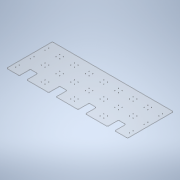
# Autodesk Inventor part: CC-bottomPlate
Saved by Autodesk Inventor 2020 (Build 240168000, 168)
## iProperties
Created: 2019-05-04
Part Number: CC-bottomPlate
Material: Polycarbonate, Clear
Document SubType Name: Modeling
Designer: andwh
Density: 1.2 g/cm^3
Appearance: Polycarbonate - Clear
Author: andwh
Autodesk Inventor part; units mm, degrees
ref_plane "YZ Plane" through (0, 0, 0) normal (1, 0, 0) x (0, 1, 0)
ref_plane "XZ Plane" through (0, 0, 0) normal (0, 1, 0) x (-1, 0, 0)
ref_plane "XY Plane" through (0, 0, 0) normal (0, 0, 1) x (1, 0, 0)
sketch "Sketch1" plane through (0, 0, 0) normal (0, 1, 0) x (-1, 0, 0)
  line L0 (0, 0) -> (-838.2, 0)
  line L1 (-838.2, 0) -> (-838.2, -317.5)
  line L2 (-838.2, -317.5) -> (0, -317.5)
  line L3 (0, -317.5) -> (0, 0)
  circle A0 centre (-63.5, -50.8) radius 44.45 construction
  circle A1 centre (-25.4, -63.5) radius 2.0193
  circle A2 centre (-101.6, -63.5) radius 2.0193
  circle A3 centre (-25.4, -38.1) radius 2.0193
  circle A4 centre (-101.6, -38.1) radius 2.0193
  circle A5 centre (-63.5, -50.8) radius 1.27 construction
  circle A6 centre (-127, -38.1) radius 2.0193
  circle A7 centre (-127, -63.5) radius 2.0193
  circle A8 centre (-165.1, -50.8) radius 1.27 construction
  circle A9 centre (-203.2, -63.5) radius 2.0193
  circle A10 centre (-203.2, -38.1) radius 2.0193
  circle A11 centre (-228.6, -38.1) radius 2.0193
  circle A12 centre (-228.6, -63.5) radius 2.0193
  circle A13 centre (-266.7, -50.8) radius 1.27 construction
  circle A14 centre (-304.8, -63.5) radius 2.0193
  circle A15 centre (-304.8, -38.1) radius 2.0193
  circle A16 centre (-330.2, -38.1) radius 2.0193
  circle A17 centre (-330.2, -63.5) radius 2.0193
  circle A18 centre (-368.3, -50.8) radius 1.27 construction
  circle A19 centre (-406.4, -63.5) radius 2.0193
  circle A20 centre (-406.4, -38.1) radius 2.0193
  circle A21 centre (-431.8, -38.1) radius 2.0193
  circle A22 centre (-431.8, -63.5) radius 2.0193
  circle A23 centre (-469.9, -50.8) radius 1.27 construction
  circle A24 centre (-508, -63.5) radius 2.0193
  circle A25 centre (-508, -38.1) radius 2.0193
  circle A26 centre (-533.4, -38.1) radius 2.0193
  circle A27 centre (-533.4, -63.5) radius 2.0193
  circle A28 centre (-571.5, -50.8) radius 1.27 construction
  circle A29 centre (-609.6, -63.5) radius 2.0193
  circle A30 centre (-609.6, -38.1) radius 2.0193
  circle A31 centre (-635, -38.1) radius 2.0193
  circle A32 centre (-635, -63.5) radius 2.0193
  circle A33 centre (-673.1, -50.8) radius 1.27 construction
  circle A34 centre (-711.2, -63.5) radius 2.0193
  circle A35 centre (-711.2, -38.1) radius 2.0193
  circle A36 centre (-736.6, -38.1) radius 2.0193
  circle A37 centre (-736.6, -63.5) radius 2.0193
  circle A38 centre (-774.7, -50.8) radius 1.27 construction
  circle A39 centre (-812.8, -63.5) radius 2.0193
  circle A40 centre (-812.8, -38.1) radius 2.0193
  circle A41 centre (-25.4, -139.7) radius 2.0193
  circle A42 centre (-25.4, -165.1) radius 2.0193
  circle A43 centre (-63.5, -152.4) radius 1.27 construction
  circle A44 centre (-101.6, -165.1) radius 2.0193
  circle A45 centre (-101.6, -139.7) radius 2.0193
  circle A46 centre (-127, -139.7) radius 2.0193
  circle A47 centre (-127, -165.1) radius 2.0193
  circle A48 centre (-165.1, -152.4) radius 1.27 construction
  circle A49 centre (-203.2, -165.1) radius 2.0193
  circle A50 centre (-203.2, -139.7) radius 2.0193
  circle A51 centre (-228.6, -139.7) radius 2.0193
  circle A52 centre (-228.6, -165.1) radius 2.0193
  circle A53 centre (-266.7, -152.4) radius 1.27 construction
  circle A54 centre (-304.8, -165.1) radius 2.0193
  circle A55 centre (-304.8, -139.7) radius 2.0193
  circle A56 centre (-330.2, -139.7) radius 2.0193
  circle A57 centre (-330.2, -165.1) radius 2.0193
  circle A58 centre (-368.3, -152.4) radius 1.27 construction
  circle A59 centre (-406.4, -165.1) radius 2.0193
  circle A60 centre (-406.4, -139.7) radius 2.0193
  circle A61 centre (-431.8, -139.7) radius 2.0193
  circle A62 centre (-431.8, -165.1) radius 2.0193
  circle A63 centre (-469.9, -152.4) radius 1.27 construction
  circle A64 centre (-508, -165.1) radius 2.0193
  circle A65 centre (-508, -139.7) radius 2.0193
  circle A66 centre (-533.4, -139.7) radius 2.0193
  circle A67 centre (-533.4, -165.1) radius 2.0193
  circle A68 centre (-571.5, -152.4) radius 1.27 construction
  circle A69 centre (-609.6, -165.1) radius 2.0193
  circle A70 centre (-609.6, -139.7) radius 2.0193
  circle A71 centre (-635, -139.7) radius 2.0193
  circle A72 centre (-635, -165.1) radius 2.0193
  circle A73 centre (-673.1, -152.4) radius 1.27 construction
  circle A74 centre (-711.2, -165.1) radius 2.0193
  circle A75 centre (-711.2, -139.7) radius 2.0193
  circle A76 centre (-736.6, -139.7) radius 2.0193
  circle A77 centre (-736.6, -165.1) radius 2.0193
  circle A78 centre (-774.7, -152.4) radius 1.27 construction
  circle A79 centre (-812.8, -165.1) radius 2.0193
  circle A80 centre (-812.8, -139.7) radius 2.0193
  circle A81 centre (-25.4, -241.3) radius 2.0193
  circle A82 centre (-25.4, -266.7) radius 2.0193
  circle A83 centre (-63.5, -254) radius 1.27 construction
  circle A84 centre (-101.6, -266.7) radius 2.0193
  circle A85 centre (-101.6, -241.3) radius 2.0193
  circle A86 centre (-127, -241.3) radius 2.0193
  circle A87 centre (-127, -266.7) radius 2.0193
  circle A88 centre (-165.1, -254) radius 1.27 construction
  circle A89 centre (-203.2, -266.7) radius 2.0193
  circle A90 centre (-203.2, -241.3) radius 2.0193
  circle A91 centre (-228.6, -241.3) radius 2.0193
  circle A92 centre (-228.6, -266.7) radius 2.0193
  circle A93 centre (-266.7, -254) radius 1.27 construction
  circle A94 centre (-304.8, -266.7) radius 2.0193
  circle A95 centre (-304.8, -241.3) radius 2.0193
  circle A96 centre (-330.2, -241.3) radius 2.0193
  circle A97 centre (-330.2, -266.7) radius 2.0193
  circle A98 centre (-368.3, -254) radius 1.27 construction
  circle A99 centre (-406.4, -266.7) radius 2.0193
  circle A100 centre (-406.4, -241.3) radius 2.0193
  circle A101 centre (-431.8, -241.3) radius 2.0193
  circle A102 centre (-431.8, -266.7) radius 2.0193
  circle A103 centre (-469.9, -254) radius 1.27 construction
  circle A104 centre (-508, -266.7) radius 2.0193
  circle A105 centre (-508, -241.3) radius 2.0193
  circle A106 centre (-533.4, -241.3) radius 2.0193
  circle A107 centre (-533.4, -266.7) radius 2.0193
  circle A108 centre (-571.5, -254) radius 1.27 construction
  circle A109 centre (-609.6, -266.7) radius 2.0193
  circle A110 centre (-609.6, -241.3) radius 2.0193
  circle A111 centre (-635, -241.3) radius 2.0193
  circle A112 centre (-635, -266.7) radius 2.0193
  circle A113 centre (-673.1, -254) radius 1.27 construction
  circle A114 centre (-711.2, -266.7) radius 2.0193
  circle A115 centre (-711.2, -241.3) radius 2.0193
  circle A116 centre (-736.6, -241.3) radius 2.0193
  circle A117 centre (-736.6, -266.7) radius 2.0193
  circle A118 centre (-774.7, -254) radius 1.27 construction
  circle A119 centre (-812.8, -266.7) radius 2.0193
  circle A120 centre (-812.8, -241.3) radius 2.0193
  dimension "d2" = 88.9
  dimension "d3" = 63.5
  dimension "d4" = 50.8
  dimension "d15" = 838.2
  dimension "d16" = 317.5
  dimension "d44" = 4.0386
  dimension "d49" = 76.2
  dimension "d52" = 25.4
  dimension "d126" = 12.7
  dimension "d127" = 38.1
  dimension "d130" = 101.6
  dimension "d133" = 101.6
  dimension "d153" = 63.5
  dimension "d154" = 2.54
  constraints: 121 centre point, 8 end point, 3 horizontal, 2 parallel, 2 vertical, 1 coincident, 1 perpendicular, 236 other
  measures "d2" diameter of A0
  measures "d3" distance from line of L3 A0.centre
  measures "d4" distance from line of L0 A0.centre
  measures "d15" distance of L1.end L2.end
  measures "d16" distance of L0.end L1.end
  measures "d44" diameter of A1
  measures "d49" distance of A1.centre A2.centre
  measures "d52" distance of A1.centre A3.centre
  measures "d126" vertical distance of A0.centre A1.centre
  measures "d127" horizontal distance of A1.centre A0.centre
  measures "d130" distance of A3.centre A6.centre
  measures "d133" distance of A3.centre A41.centre
  measures "d153" distance from line of L2 A83.centre
  measures "d154" diameter of A5
extrude "Extrusion1" add sketch "Sketch1" against normal blind 3.175
sketch "Sketch5" plane through (0, 0, 0) normal (0, 1, 0) x (1, 0, 0)
  line L0 (838.2, 0) -> (0, 0) projected
  line L1 (88.9, 0) -> (139.7, 0)
  line L2 (139.7, 0) -> (139.7, 76.2)
  line L3 (139.7, 76.2) -> (88.9, 76.2)
  line L4 (88.9, 76.2) -> (88.9, 0)
  circle A0 centre (101.6, 63.5) radius 2.0193 projected
  circle A1 centre (127, 63.5) radius 2.0193 projected
  line L5 (292.1, 76.2) -> (292.1, 0)
  line L6 (342.9, 76.2) -> (292.1, 76.2)
  line L7 (342.9, 0) -> (342.9, 76.2)
  line L8 (292.1, 0) -> (342.9, 0)
  line L9 (495.3, 76.2) -> (495.3, 0)
  line L10 (546.1, 76.2) -> (495.3, 76.2)
  line L11 (546.1, 0) -> (546.1, 76.2)
  line L12 (495.3, 0) -> (546.1, 0)
  line L13 (698.5, 76.2) -> (698.5, 0)
  line L14 (749.3, 76.2) -> (698.5, 76.2)
  line L15 (749.3, 0) -> (749.3, 76.2)
  line L16 (698.5, 0) -> (749.3, 0)
  dimension "d155" = 12.7
  dimension "d156" = 12.7
  dimension "d157" = 12.7
  dimension "d160" = 203.2
  constraints: 32 end point, 2 horizontal, 2 parallel, 1 perpendicular, 1 point on line, 24 other
  measures "d155" distance from line of L3 A0.centre
  measures "d156" distance from line of L4 A0.centre
  measures "d157" distance from line of L2 A1.centre
  measures "d160" distance of L3.end L5.start
extrude "Extrusion4" cut sketch "Sketch5" against normal through all
fillet "Fillet1" radius 6.35 20 edges at (0, -1.5875, 0) (838.2, -1.5875, 0) (838.2, -1.5875, -317.5) (0, -1.5875, -317.5) (749.3, -1.5875, -76.2) (698.5, -1.5875, -76.2) (546.1, -1.5875, -76.2) (495.3, -1.5875, -76.2) (88.9, -1.5875, -76.2) (139.7, -1.5875, -76.2) (342.9, -1.5875, -76.2) (292.1, -1.5875, -76.2) (88.9, -1.5875, 0) (139.7, -1.5875, 0) (342.9, -1.5875, 0) (292.1, -1.5875, 0) (495.3, -1.5875, 0) (546.1, -1.5875, 0) (698.5, -1.5875, 0) (749.3, -1.5875, 0)
body "Solid1"
